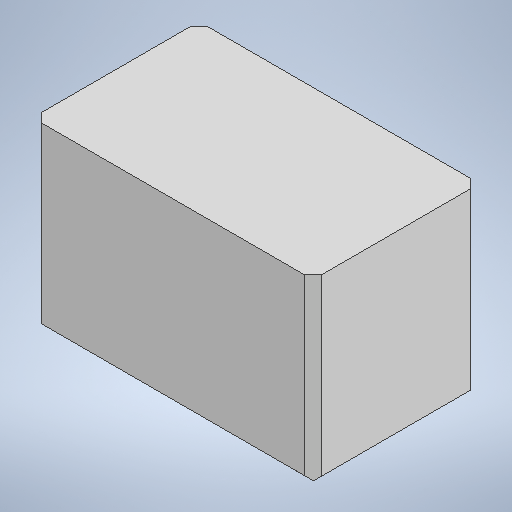
# Autodesk Inventor part: GBK-RK-0005 RK dummy 5
Saved by Autodesk Inventor 2026.2 (Build 302298000, 298)
## iProperties
allow_slope_adjustment: 0 ul
flow_configuration2: 1 ul
flow_direction: 2 ul
loss_method: 0 ul
radius: 162,500 mm
Created: 2026-08-26
Part Number: GBK-RK-0005 RK dummy 5
Material: Water
Document SubType Name: Modeling
Designer: admin
Mass: 5.80711e+06 g
Surface Area: 199540 cm^2
Volume: 5.817e+06 cm^3
Density: 0.9983 g/cm^3
Appearance: Default
radius: 200,000 mm
Author: admin
Autodesk Inventor part; units mm, degrees
ref_plane "YZ Plane" through (0, 0, 0) normal (1, 0, 0) x (0, 1, 0)
ref_plane "XZ Plane" through (0, 0, 0) normal (0, 1, 0) x (-1, 0, 0)
ref_plane "XY Plane" through (0, 0, 0) normal (0, 0, 1) x (1, 0, 0)
sketch "Sketch18" plane through (0, 0, 0) normal (0, 0, 1) x (1, 0, 0)
  circle A0 centre (0, 1100) radius 213
  line L0 (0, 0) -> (0, 1100) construction
  line L1 (0, 1100) -> (0, 1600) construction
  line L2 (0, 1100) -> (-158.3548, 850) construction
  line L3 (-158.3548, 850) -> (-454.2876, 850) construction
  line L4 (-454.2876, 850) -> (-612.6424, 1100) construction
  line L5 (-612.6424, 1100) -> (0, 1100) construction
  line L6 (-1230, 1600) -> (1230, 1600)
  line L7 (1541.1151, -621.787) -> (-1872.5331, -621.787) construction
  line L8 (-1230, 1600) -> (-1230, 265.165)
  line L9 (-1230, 265.165) -> (-964.835, 0)
  line L10 (-964.835, 0) -> (1159.2893, 0)
  line L11 (1159.2893, 0) -> (1230, 70.7107)
  line L12 (1230, 70.7107) -> (1230, 1600)
  line L13 (-1468.3883, 141.4214) -> (-1468.3883, -183.5786)
  line L14 (-1468.3883, 198.9214) -> (-1496.3883, 198.9214)
  line L15 (-1496.3883, 198.9214) -> (-1496.3883, -241.0786)
  line L16 (-1496.3883, -241.0786) -> (-1468.3883, -241.0786)
  line L17 (-1468.3883, -241.0786) -> (-1468.3883, 198.9214)
  line L18 (-1097.4175, 132.5825) -> (-1251.0786, -21.0786) construction
  line L19 (-1251.0786, -21.0786) -> (-1468.3883, -21.0786) construction
  line L20 (-1468.3883, 141.4214) -> (-1318.3883, 141.4214)
  line L21 (-1318.3883, 141.4214) -> (-1212.3223, 247.4874)
  line L22 (-1468.3883, -183.5786) -> (-1183.7689, -183.5786)
  line L23 (-1183.7689, -183.5786) -> (-982.5126, 17.6777)
  line L24 (-1318.3883, 141.4214) -> (-1183.7689, -183.5786)
  line L25 (1313.2107, -113.2107) -> (1341.2107, -113.2107)
  line L26 (1341.2107, -113.2107) -> (1341.2107, -553.2107)
  line L27 (1341.2107, -553.2107) -> (1313.2107, -553.2107)
  line L28 (1313.2107, -553.2107) -> (1313.2107, -113.2107)
  line L29 (980, 0) -> (980, -135.3553) construction
  line L30 (980, -135.3553) -> (1177.8553, -333.2107) construction
  line L31 (1177.8553, -333.2107) -> (1313.2107, -333.2107) construction
  line L32 (1313.2107, -170.7107) -> (1213.2107, -170.7107)
  line L33 (1213.2107, -170.7107) -> (1142.5, -100)
  line L34 (1142.5, -100) -> (1142.5, 0)
  line L35 (1313.2107, -495.7107) -> (1142.5, -495.7107)
  line L36 (1142.5, -495.7107) -> (817.5, -170.7107)
  line L37 (817.5, -170.7107) -> (817.5, 0)
  line L38 (1142.5, -100) -> (817.5, -170.7107)
  line L39 (1213.2107, -170.7107) -> (1142.5, -495.7107)
  line L40 (1177.8553, -135.3553) -> (980, -333.2107) construction
  line L41 (1142.5, -50) -> (817.5, -50) construction
  line L42 (-764.544, 0) -> (-593.6658, 0)
  line L43 (28, 0) -> (23.8247, 0)
  line L44 (28, -50) -> (28, 0)
  line L45 (28, -50) -> (-28, -50)
  line L46 (-28, -50) -> (-28, -22)
  line L47 (-28, -22) -> (0, -22)
  line L48 (0, -22) -> (0, 0)
  line L49 (0, -22) -> (28, -22) construction
  line L50 (-33.8617, -50) -> (33.8617, -50)
  line L51 (33.8617, -50) -> (33.8617, -60)
  line L52 (33.8617, -60) -> (-33.8617, -60)
  line L53 (-33.8617, -60) -> (-33.8617, -50)
  line L54 (-37.5, -60) -> (37.5, -60)
  line L55 (37.5, -60) -> (37.5, -200)
  line L56 (37.5, -200) -> (-37.5, -200)
  line L57 (-37.5, -200) -> (-37.5, -60)
  line L58 (378, 0) -> (373.8247, 0)
  line L59 (350, -22) -> (350, 0)
  line L60 (322, -22) -> (350, -22)
  line L61 (350, -22) -> (378, -22) construction
  line L62 (322, -50) -> (322, -22)
  line L63 (378, -50) -> (378, 0)
  line L64 (378, -50) -> (322, -50)
  line L65 (387.5, -60) -> (387.5, -200)
  line L66 (383.8617, -50) -> (383.8617, -60)
  line L67 (312.5, -200) -> (312.5, -60)
  line L68 (387.5, -200) -> (312.5, -200)
  line L69 (316.1383, -50) -> (383.8617, -50)
  line L70 (383.8617, -60) -> (316.1383, -60)
  line L71 (312.5, -60) -> (387.5, -60)
  line L72 (316.1383, -60) -> (316.1383, -50)
  line L73 (-322, 0) -> (-326.1753, 0)
  line L74 (-350, -22) -> (-350, 0)
  line L75 (-378, -22) -> (-350, -22)
  line L76 (-350, -22) -> (-322, -22) construction
  line L77 (-378, -50) -> (-378, -22)
  line L78 (-322, -50) -> (-322, 0)
  line L79 (-322, -50) -> (-378, -50)
  line L80 (-312.5, -60) -> (-312.5, -200)
  line L81 (-316.1383, -50) -> (-316.1383, -60)
  line L82 (-387.5, -200) -> (-387.5, -60)
  line L83 (-312.5, -200) -> (-387.5, -200)
  line L84 (-383.8617, -50) -> (-316.1383, -50)
  line L85 (-316.1383, -60) -> (-383.8617, -60)
  line L86 (-387.5, -60) -> (-312.5, -60)
  line L87 (-383.8617, -60) -> (-383.8617, -50)
  line L88 (728, 0) -> (723.8247, 0)
  line L89 (700, -22) -> (700, 0)
  line L90 (672, -22) -> (700, -22)
  line L91 (700, -22) -> (728, -22) construction
  line L92 (672, -50) -> (672, -22)
  line L93 (728, -50) -> (728, 0)
  line L94 (728, -50) -> (672, -50)
  line L95 (737.5, -60) -> (737.5, -200)
  line L96 (733.8617, -50) -> (733.8617, -60)
  line L97 (662.5, -200) -> (662.5, -60)
  line L98 (737.5, -200) -> (662.5, -200)
  line L99 (666.1383, -50) -> (733.8617, -50)
  line L100 (733.8617, -60) -> (666.1383, -60)
  line L101 (662.5, -60) -> (737.5, -60)
  line L102 (666.1383, -60) -> (666.1383, -50)
  line L103 (-672, 0) -> (-676.1753, 0)
  line L104 (-700, -22) -> (-700, 0)
  line L105 (-728, -22) -> (-700, -22)
  line L106 (-700, -22) -> (-672, -22) construction
  line L107 (-728, -50) -> (-728, -22)
  line L108 (-672, -50) -> (-672, 0)
  line L109 (-672, -50) -> (-728, -50)
  line L110 (-662.5, -60) -> (-662.5, -200)
  line L111 (-666.1383, -50) -> (-666.1383, -60)
  line L112 (-737.5, -200) -> (-737.5, -60)
  line L113 (-662.5, -200) -> (-737.5, -200)
  line L114 (-733.8617, -50) -> (-666.1383, -50)
  line L115 (-666.1383, -60) -> (-733.8617, -60)
  line L116 (-737.5, -60) -> (-662.5, -60)
  line L117 (-733.8617, -60) -> (-733.8617, -50)
  line L118 (-1230, 265.165) -> (-1230, 70.7107)
  line L119 (-1230, 70.7107) -> (-1159.2893, 0)
  line L120 (-1159.2893, 0) -> (-964.835, 0)
  line L121 (1980.1647, -124.622) -> (1655.1647, -124.622)
  line L122 (1655.1647, -124.622) -> (1655.1647, -361.6901)
  line L123 (2165.0175, -309.4748) -> (2165.0175, -634.4748)
  line L124 (1980.1647, -124.622) -> (1980.1647, -309.4748)
  line L125 (1980.1647, -309.4748) -> (2165.0175, -309.4748)
  line L126 (2022.5911, -267.0484) -> (1791.5571, -498.0824)
  line L127 (1980.1647, -224.622) -> (2065.0175, -309.4748)
  line L128 (1655.1647, -361.6901) -> (1927.9494, -634.4748)
  line L129 (1980.1647, -224.622) -> (1655.1647, -361.6901)
  line L130 (2065.0175, -309.4748) -> (1927.9494, -634.4748)
  line L131 (2165.0175, -634.4748) -> (1927.9494, -634.4748)
  point P0 (-306.3212, 850)
  point P1 (-306.3212, 1100)
  point P2 (0, -50)
  point P3 (0, -60)
  point P4 (350, 0)
  point P5 (350, -50)
  point P6 (350, -60)
  point P7 (-350, 0)
  point P8 (-350, -50)
  point P9 (-350, -60)
  point P10 (700, 0)
  point P11 (700, -50)
  point P12 (700, -60)
  point P13 (-700, 0)
  point P14 (-700, -50)
  point P15 (-700, -60)
  dimension "d112" = 426
  dimension "d113" = 1100
  dimension "d114" = 500
  dimension "d115" = 1100
  dimension "d116" = 250
  dimension "d120" = 2460
  dimension "d121" = 325
  dimension "d123" = 28
  dimension "d124" = 440
  dimension "d125" = 135
  dimension "d127" = 67.5
  dimension "d128" = 100
  dimension "d129" = 375
  dimension "d130" = 1600
  dimension "d131" = 150
  dimension "d132" = 250
  dimension "d133" = 100
  dimension "d135" = 50
  dimension "d136" = -28
  dimension "d137" = 10
  dimension "d138" = 140
  dimension "d139" = 75
  dimension "d142" = 350
  dimension "d157" = 217.3097
  dimension "d164" = 135.3553
  dimension "d165" = 279.8097
  dimension "d174" = 12.275
  dimension "d175" = 32.725
  dimension "d176" = 459.6194
  dimension "d177" = 279.8097
  dimension "d178" = 325
  dimension "d179" = 45
  dimension "d180" = 100
  dimension "d181" = 100
  dimension "d182" = 120
  dimension "d184" = 326.7315
  dimension "d185" = 22.867
  dimension "d186" = 22.133
  constraints: 264 end point, 24 perpendicular, 21 point on line, 19 midpoint, 18 horizontal, 12 equal length, 11 parallel, 8 vertical, 1 centre point, 1 coincident, 1 collinear, 1 vertical alignment, 138 other
  measures "d112" diameter of A0
  measures "d113" distance of L0.start L0.end
  measures "d114" distance of L1.end L0.end
  measures "d115" distance of L0.start A0.centre
  measures "d116" distance between parallel lines of L3 L5
  measures "d120" distance of L6.start L6.end
  measures "d121" distance of L13.start L13.end
  measures "d123" distance of L16.end L15.end
  measures "d124" distance of L15.end L14.end
  measures "d125" angle of L9 L8
  measures "d127" angle of L23 L24
  measures "d128" distance of L10.end L11.end
  measures "d129" distance of L8.end L9.end
  measures "d130" distance between parallel lines of L10 L6
  measures "d131" distance of L20.end L21.end
  measures "d132" distance between parallel lines of L12 L29
  measures "d133" distance of L33.end L34.end
  measures "d135" distance of L44.start L43.start
  measures "d136" distance between parallel lines of L0 L44
  measures "d137" distance of L52.end L50.start
  measures "d138" distance of L56.end L54.start
  measures "d139" distance of L55.end L56.end
  measures "d142" distance of L0.start point (350, 0)
  measures "d157" distance of L18.end L19.end
  measures "d164" distance of L30.end L31.end
  measures "d165" distance of L29.end L30.end
  measures "d174" angle of L41 L38
  measures "d175" angle of L38 L40
  measures "d176" distance of L35.end L36.end
  measures "d177" distance of L40.start L40.end
  measures "d178" distance of L121.start L121.end
  measures "d179" angle of L126 L121
  measures "d180" distance of L127.start L121.start
  measures "d181" distance of L123.start L127.end
  measures "d182" distance of L127.start L127.end
  measures "d184" distance between parallel lines of L128 L127
  measures "d185" angle of L129 L121
  measures "d186" angle of L126 L129
extrude "Extrusion16" add sketch "Sketch18" along normal mid plane 1460 contours A0 | L6 L12 L11 L10 L9 L8 | L9 L21 L118 | L9 L23 L120 L119 L118 L21 | L9 L120 L23
sketch "Sketch19" plane through (-1230, 265.165, 700) normal (-1, 0, 0) x (0, 0, 1)
  circle A0 centre (-700, 834.835) radius 213
  line L0 (30, 1334.835) -> (30, -194.4544) construction
  line L1 (-1430, 1334.835) -> (30, 1334.835) construction
  line L2 (-1430, -194.4544) -> (-1430, 1334.835) construction
  line L3 (-1430, 1334.835) -> (30, 1334.835) projected
  line L4 (-1430, -194.4544) -> (30, -194.4544) projected
  point P0 (-700, -265.165)
  point P1 (-700, 1334.835)
  point P2 (-700, 1334.835)
  dimension "d149" = 500
  dimension "d150" = 426
  constraints: 2 midpoint, 1 centre point, 1 vertical alignment
  measures "d149" distance of A0.centre point (-700, 1334.835)
  measures "d150" diameter of A0
extrude "Extrusion17" [suppressed]
sketch "Sketch20" plane through (0, 0, -730) normal (0, 0, -1) x (-1, 0, 0)
  circle A0 centre (0, 1100) radius 213
  line L0 (1230, 1600) -> (-1230, 1600) projected
  point P0 (0, 0)
  point P1 (0, 1600)
  point P2 (0, 1600)
  dimension "d153" = 500
  dimension "d154" = 426
  constraints: 2 midpoint, 1 centre point, 1 vertical alignment
  measures "d153" distance of point (0, 1600) A0.centre
  measures "d154" diameter of A0
extrude "Extrusion18" [suppressed]
sketch "Sketch23" plane through (0, 0, 0) normal (0, 0, 1) x (1, 0, 0)
  line L0 (1159.2893, 0) -> (1230, 70.7107) construction
  line L1 (1230, 70.7107) -> (1230, 1600) construction
  line L2 (1230, 1600) -> (-1230, 1600) construction
  line L3 (-1230, 1600) -> (-1230, 70.7107) construction
  line L4 (980, 0) -> (980, -135.3553)
  line L5 (980, -135.3553) -> (1177.8553, -333.2107)
  line L6 (1177.8553, -333.2107) -> (1313.2107, -333.2107)
  line L7 (-1159.2893, 0) -> (1159.2893, 0) projected
  line L8 (-1230, 70.7107) -> (-1159.2893, 0) projected
  point P0 (0, 0)
  dimension "d162" = 135
  dimension "d163" = 250
  dimension "d166" = 135.3553
  dimension "d167" = 279.8097
  constraints: 6 end point, 2 perpendicular
  measures "d162" angle of L5 L4
  measures "d163" distance between parallel lines of L1 L4
  measures "d166" distance of L4.start L4.end
  measures "d167" distance of L4.end L5.end
sketch "Sketch24" plane through (-1034.835, 0, 700) normal (0, -1, 0) x (1, 0, 0)
  circle A0 centre (2084.835, -700) radius 162.5
  point P0 (1034.835, -700)
  dimension "d168" = 325
  constraints: 1 centre point, 1 coincident
  measures "d168" diameter of A0
sweep "Sweep4" [suppressed]
mirror "Mirror7" [suppressed]
mirror "Mirror8" [suppressed]
chamfer "Chamfer2" distance 75 angle 45 6 edges at (-1230, 835.3553, 730) (0, 0, 730) (1230, 835.3553, 730) (1230, 835.3553, -730) (0, 0, -730) (-1230, 835.3553, -730)
body "Solid2"
